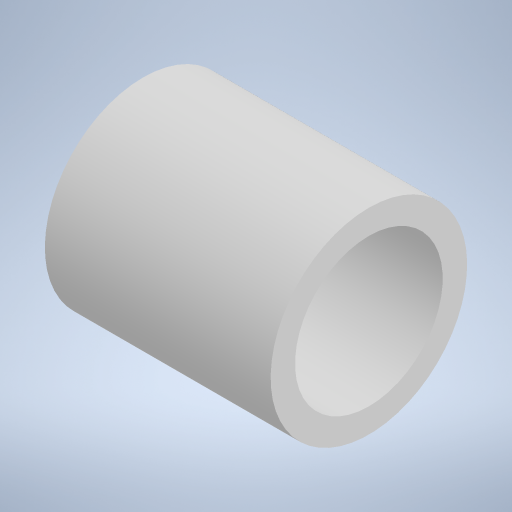
# Autodesk Inventor part: 18.5mmSpacer
Saved by Autodesk Inventor 2023 (Build 270158000, 158)
## iProperties
Created: 2022-09-23
Part Number: 18.5mmSpacer
Material: Generic
Document SubType Name: Modeling
Designer: deli
Density: 1 g/cm^3
Appearance: Default
Author: deli
Autodesk Inventor part; units mm, degrees
ref_plane "YZ Plane" through (0, 0, 0) normal (1, 0, 0) x (0, 1, 0)
ref_plane "XZ Plane" through (0, 0, 0) normal (0, 1, 0) x (-1, 0, 0)
ref_plane "XY Plane" through (0, 0, 0) normal (0, 0, 1) x (1, 0, 0)
sketch "Sketch1" plane through (0, 0, 0) normal (1, 0, 0) x (0, 1, 0)
  circle A0 centre (-1.0156, 62.6937) radius 8.05 projected
  circle A1 centre (-1.0156, 62.6937) radius 6.05 projected
  point P0 (0, 0)
extrude "Extrusion1" add sketch "Sketch1" along normal blind 18.5
body "Solid1"
